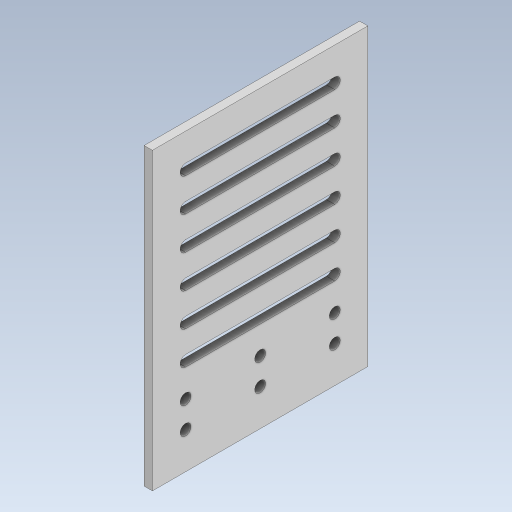
# Autodesk Inventor part: Wall Conyevor Kiri
Saved by Autodesk Inventor 2023.5 (Build 275446000, 446)
## iProperties
Created: 2025-10-12
Part Number: Wall Conyevor Kiri
Material: Generic
Document SubType Name: Modeling
Designer: Guntur
Density: 1 g/cm^3
Appearance: Default
Author: Guntur
## iProperties of the stored document Wall Conyevor Belakang_3DPrint.ipt
Created: 2025-10-20
Part Number: Wall Conyevor Belakang_3DPrint
Material: Generic
Document SubType Name: Modeling
Designer: Guntur
Density: 1 g/cm^3
Appearance: Default
Author: Guntur
Autodesk Inventor part; units mm, degrees
ref_plane "YZ Plane" through (0, 0, 0) normal (1, 0, 0) x (0, 1, 0)
ref_plane "XZ Plane" through (0, 0, 0) normal (0, 1, 0) x (-1, 0, 0)
ref_plane "XY Plane" through (0, 0, 0) normal (0, 0, 1) x (1, 0, 0)
sketch "Sketch1" plane through (0, 0, 0) normal (1, 0, 0) x (0, 1, 0)
  circle A0 centre (0, 0) radius 1.65
  circle A1 centre (0, -22.5) radius 1.65
  line L0 (34, 0) -> (-44, 0) construction
  line L1 (0, 41) -> (0, -59) construction
  circle A2 centre (-8, 0) radius 1.65
  circle A3 centre (0, 22.5) radius 1.65
  line L2 (-19, -22.5) -> (-19, 22.5)
  line L3 (0, 22.5) -> (0, -22.5)
  line L4 (-19, -22.5) -> (-19, -32.5)
  line L5 (-19, -32.5) -> (0, -32.5)
  line L6 (0, -32.5) -> (0, -22.5)
  line L7 (-19, 22.5) -> (-19, 32.5)
  line L8 (-19, 32.5) -> (0, 32.5)
  line L9 (0, 32.5) -> (0, 22.5)
  line L10 (0, -32.5) -> (70, -32.5)
  line L11 (70, -32.5) -> (70, 32.5)
  line L12 (70, 32.5) -> (0, 32.5)
  line L13 (0, 32.5) -> (0, -32.5)
  circle A4 centre (-8, -22.5) radius 1.65
  circle A5 centre (-8, 22.5) radius 1.65
  circle A6 centre (10, -22.5) radius 1.65
  circle A7 centre (10, 22.5) radius 1.65
  line L14 (10, -22.5) -> (10, 22.5) construction
  line L15 (11.65, -22.5) -> (11.65, 22.5)
  line L16 (8.35, 22.5) -> (8.35, -22.5)
  arc A8 (8.35, -22.5) -> (11.65, -22.5) centre (10, -22.5) ccw
  arc A9 (11.65, 22.5) -> (8.35, 22.5) centre (10, 22.5) ccw
  line L17 (18.35, 22.5) -> (18.35, -22.5)
  line L18 (20, -22.5) -> (20, 22.5) construction
  line L19 (21.65, -22.5) -> (21.65, 22.5)
  arc A10 (21.65, 22.5) -> (18.35, 22.5) centre (20, 22.5) ccw
  circle A11 centre (20, 22.5) radius 1.65
  circle A12 centre (20, -22.5) radius 1.65
  arc A13 (18.35, -22.5) -> (21.65, -22.5) centre (20, -22.5) ccw
  line L20 (28.35, 22.5) -> (28.35, -22.5)
  line L21 (30, -22.5) -> (30, 22.5) construction
  line L22 (31.65, -22.5) -> (31.65, 22.5)
  arc A14 (31.65, 22.5) -> (28.35, 22.5) centre (30, 22.5) ccw
  circle A15 centre (30, 22.5) radius 1.65
  circle A16 centre (30, -22.5) radius 1.65
  arc A17 (28.35, -22.5) -> (31.65, -22.5) centre (30, -22.5) ccw
  line L23 (38.35, 22.5) -> (38.35, -22.5)
  line L24 (40, -22.5) -> (40, 22.5) construction
  line L25 (41.65, -22.5) -> (41.65, 22.5)
  arc A18 (41.65, 22.5) -> (38.35, 22.5) centre (40, 22.5) ccw
  circle A19 centre (40, 22.5) radius 1.65
  circle A20 centre (40, -22.5) radius 1.65
  arc A21 (38.35, -22.5) -> (41.65, -22.5) centre (40, -22.5) ccw
  line L26 (48.35, 22.5) -> (48.35, -22.5)
  line L27 (50, -22.5) -> (50, 22.5) construction
  line L28 (51.65, -22.5) -> (51.65, 22.5)
  arc A22 (51.65, 22.5) -> (48.35, 22.5) centre (50, 22.5) ccw
  circle A23 centre (50, 22.5) radius 1.65
  circle A24 centre (50, -22.5) radius 1.65
  arc A25 (48.35, -22.5) -> (51.65, -22.5) centre (50, -22.5) ccw
  line L29 (58.35, 22.5) -> (58.35, -22.5)
  line L30 (60, -22.5) -> (60, 22.5) construction
  line L31 (61.65, -22.5) -> (61.65, 22.5)
  arc A26 (61.65, 22.5) -> (58.35, 22.5) centre (60, 22.5) ccw
  circle A27 centre (60, 22.5) radius 1.65
  circle A28 centre (60, -22.5) radius 1.65
  arc A29 (58.35, -22.5) -> (61.65, -22.5) centre (60, -22.5) ccw
  point P0 (0, -1.34)
  point P1 (0, 32.5)
  point P2 (0, 0)
  point P3 (10, 0)
  point P4 (20, 0)
  point P5 (30, 0)
  point P6 (40, 0)
  point P7 (50, 0)
  point P8 (60, 0)
  point P9 (21.65, -22.5)
  dimension "d0" = 3.3
  dimension "d1" = 3.3
  dimension "d5" = 3.3
  dimension "d22" = 10
  dimension "d23" = 10
  dimension "d24" = 22.5
  dimension "d25" = 22.5
  dimension "d26" = 3.3
  dimension "d27" = 3.3
  dimension "d30" = 70
  dimension "d31" = 3.3
  dimension "d32" = 10
  dimension "d33" = 3.3
  dimension "d36" = 10
  constraints: 76 end point, 30 centre point, 24 point on circle, 6 parallel, 4 horizontal, 4 tangent, 3 vertical, 2 midpoint, 2 point on line, 1 coincident, 1 concentric, 1 perpendicular, 1 symmetric about line, 71 other
  measures "d0" diameter of A0
  measures "d1" diameter of A1
  measures "d5" diameter of A2
  measures "d22" distance of L4.end L4.start
  measures "d23" distance of L7.start L7.end
  measures "d24" distance of point (0, 0) L3.end
  measures "d25" distance of point (0, 0) A3.centre
  measures "d26" diameter of A4
  measures "d27" diameter of A5
  measures "d30" distance of L11.end L12.end
  measures "d31" diameter of A6
  measures "d32" distance of L3.end L14.start
  measures "d33" diameter of A7
  measures "d36" distance of L16.start L17.start
extrude "Extrusion2" add sketch "Sketch1" along normal blind 2.5 contours A0 L3 A3 L9 L12 L11 L10 L6 A1 | A0 L3 A1 L6 L5 L4 L2 L7 L8 L9 A3
body "Solid2"
